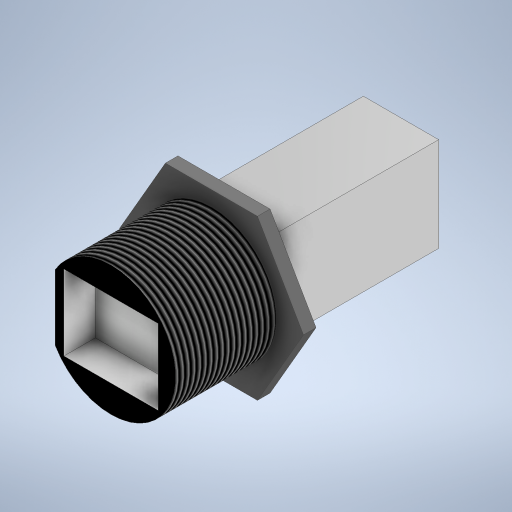
# Autodesk Inventor part: RS PRO Single-Port RJ45 Female Coupler, Shielded
Saved by Autodesk Inventor 2023 (Build 270158000, 158)
## iProperties
Created: 2023-04-24
Part Number: RS PRO Single-Port RJ45 Female Coupler, Shielded
Material: Generic
Document SubType Name: Modeling
Designer: Louis
Density: 1 g/cm^3
Appearance: Default
Author: Louis
Autodesk Inventor part; units mm, degrees
ref_plane "YZ Plane" through (0, 0, 0) normal (1, 0, 0) x (0, 1, 0)
ref_plane "XZ Plane" through (0, 0, 0) normal (0, 1, 0) x (-1, 0, 0)
ref_plane "XY Plane" through (0, 0, 0) normal (0, 0, 1) x (1, 0, 0)
sketch "Sketch1" plane through (0, 0, 0) normal (0, 0, 1) x (1, 0, 0)
  circle A0 centre (0, 0) radius 10.3188
  line L0 (-8.8812, 5.2536) -> (-8.8812, -5.2536)
  dimension "d0" = 20.6375
  dimension "d10" = 19.2
  constraints: 2 end point, 2 point on circle, 1 centre point, 1 coincident, 1 vertical
  measures "d0" diameter of A0
extrude "Extrusion1" add sketch "Sketch1" along normal blind 16 contours A0 L0 picked at (-2.4812, 0)
sketch "Sketch2" plane through (0, 0, 0) normal (0, 0, -1) x (0, -1, 0)
  line L0 (0, 14.6647) -> (12.7, 7.3323)
  line L1 (12.7, 7.3323) -> (12.7, -7.3323)
  line L2 (12.7, -7.3323) -> (0, -14.6647)
  line L3 (0, -14.6647) -> (-12.7, -7.3323)
  line L4 (-12.7, -7.3323) -> (-12.7, 7.3323)
  line L5 (-12.7, 7.3323) -> (0, 14.6647)
  point P0 (0, 0)
  point P1 (0, 0)
  dimension "d3" = 25.4
  constraints: 12 end point, 1 coincident, 13 other
  measures "d3" distance between parallel lines of L1 L4
extrude "Extrusion2" add sketch "Sketch2" along normal blind 2
sketch "Sketch3" plane through (0, 0, -2) normal (0, 0, -1) x (0, -1, 0)
  line L0 (-7.5, 6) -> (7.5, 6)
  line L1 (7.5, 6) -> (7.5, -6)
  line L2 (7.5, -6) -> (-7.5, -6)
  line L3 (-7.5, -6) -> (-7.5, 6)
  point P0 (0, 0)
  point P1 (-7.5, 0)
  point P2 (0, 6)
  dimension "d6" = 15
  dimension "d7" = 12
  constraints: 8 end point, 2 midpoint, 2 parallel, 1 horizontal, 1 horizontal alignment, 1 perpendicular, 1 vertical alignment
  measures "d6" distance of L0.start L0.end
  measures "d7" distance of L0.end L1.end
extrude "Extrusion3" add sketch "Sketch3" along normal blind 28.2
thread "Thread1" size "13/16-28 UN" class "2A" standard "ANSI Unified Screw Threads" full length
sketch "Sketch4" plane through (0, 0, 16) normal (0, 0, 1) x (1, 0, 0)
  line L0 (-7.5, 6) -> (7.5, 6)
  line L1 (7.5, 6) -> (7.5, -6)
  line L2 (7.5, -6) -> (-7.5, -6)
  line L3 (-7.5, -6) -> (-7.5, 6)
  point P0 (0, 0)
  point P1 (7.5, 0)
  point P2 (0, 6)
  dimension "d13" = 15
  dimension "d14" = 12
  constraints: 8 end point, 2 midpoint, 2 parallel, 1 horizontal, 1 horizontal alignment, 1 perpendicular, 1 vertical alignment
  measures "d13" distance of L0.start L0.end
  measures "d14" distance of L0.end L1.end
extrude "Extrusion4" cut sketch "Sketch4" against normal blind 5
body "Solid1"
